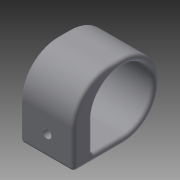
# Autodesk Inventor part: LoopD
Saved by Autodesk Inventor 2014 (Build 180170000, 170)
## iProperties
Created: 2014-06-16
Part Number: LoopD
Material: Generisch
Document SubType Name: Modeling
Designer: g.schardt
Density: 1 g/cm^3
Appearance: Vorgabe
Author: g.schardt
Autodesk Inventor part; units mm, degrees
ref_plane "YZ Plane" through (0, 0, 0) normal (1, 0, 0) x (0, 1, 0)
ref_plane "XZ Plane" through (0, 0, 0) normal (0, 1, 0) x (-1, 0, 0)
ref_plane "XY Plane" through (0, 0, 0) normal (0, 0, 1) x (1, 0, 0)
sketch "Skizze1" plane through (0, 0, 0) normal (1, 0, 0) x (0, 1, 0)
  line L0 (-21, -18) -> (21, -18)
  line L1 (21, -18) -> (21, 18)
  line L2 (21, 18) -> (-21, 18)
  line L3 (-21, 18) -> (-21, -18)
  line L4 (-21, -18) -> (21, 18) construction
  line L5 (21, -18) -> (-21, 18) construction
  point P0 (0, 0)
  dimension "d0" = 42
  dimension "d1" = 36
  constraints: 12 end point, 2 midpoint, 2 parallel, 1 horizontal, 1 perpendicular
  measures "d0" distance of L2.end L1.end
  measures "d1" distance of L1.end L0.end
extrude "Extrusion1" add sketch "Skizze1" along normal blind 26
sketch "Skizze2" plane through (26, 0, 0) normal (1, 0, 0) x (0, 0, -1)
  line L0 (18, 21) -> (-18, 21) projected
  line L1 (-18, 21) -> (-18, -21) projected
  line L2 (-15, 18) -> (15, 18)
  line L3 (15, 18) -> (15, -12)
  line L4 (15, -12) -> (-15, -12)
  line L5 (-15, -12) -> (-15, 18)
  point P0 (0, 0)
  dimension "d4" = 30
  dimension "d5" = 30
  dimension "d6" = 3
  dimension "d7" = 3
  constraints: 8 end point, 2 parallel, 1 horizontal, 1 perpendicular
  measures "d4" distance of L2.start L2.end
  measures "d5" distance between parallel lines of L4 L2
  measures "d6" distance between parallel lines of L0 L2
  measures "d7" distance between parallel lines of L1 L5
extrude "Extrusion2" cut sketch "Skizze2" against normal through all
fillet "Rundung1" radius 15 1 edges at (13, 18, -15)
fillet "Rundung2" radius 15 1 edges at (13, 18, 15)
fillet "Rundung3" radius 18 2 edges at (13, 21, 18) (13, 21, -18)
ref_plane "Arbeitsebene1" through (0, -18, -18) normal (0, -1, 0) x (1, 0, 0)
ref_plane "Arbeitsebene2" through (0, -14.8, -18) normal (0, -1, 0) x (1, 0, 0)
sketch "Skizze3" plane through (0, -21, -18) normal (0, -1, 0) x (1, 0, 0)
  line L0 (0, 36) -> (0, 0) projected
  line L1 (0, 0) -> (26, 0) projected
  line L2 (3, 0) -> (23, 0)
  line L3 (23, 0) -> (23, 17)
  line L4 (23, 17) -> (3, 17)
  line L5 (3, 17) -> (3, 0)
  point P0 (0, 18)
  dimension "d15" = 20
  dimension "d16" = 17
  dimension "d17" = 3
  constraints: 8 end point, 2 parallel, 1 horizontal, 1 perpendicular, 1 point on line
  measures "d15" distance of L4.end L3.end
  measures "d16" distance of L3.end L2.end
  measures "d17" distance between parallel lines of L0 L5
extrude "Extrusion3" cut sketch "Skizze3" against normal up to surface (3.2 mm away) from surface at -3
fillet "Rundung4" radius 9 2 edges at (3, -16.4, -1) (23, -16.4, -1)
sketch "Skizze4" plane through (26, -12, 15) normal (0, 1, 0) x (1, 0, 0)
  line L0 (0, 30) -> (0, 0) projected
  line L1 (-26, -3) -> (0, -3) projected
  line L2 (-3, 33) -> (-23, 33) projected
  point P0 (-26, 15)
  point P1 (-13, 23)
  dimension "d29" = 13
  dimension "d31" = 10
  measures "d29" distance from line of L0 point (-13, 23)
  measures "d31" distance from line of L2 point (-13, 23)
hole "Bohrung1" at (13, -12, -8) direction (0, -1, 0) diameter 4.2 end through all countersink diameter 7.5 countersink angle 90
fillet "Rundung10" radius 15 1 edges at (13, -12, 15)
fillet "Rundung11" radius 18 1 edges at (13, -21, 18)
fillet "Rundung12" radius 1.5 29 edges at (26, -8.9999, -18) (26, 0, 18) (26, -15.7279, 12.7279) (26, -21, -9) (26, 15.728, 12.728) (26, 21, 0) (26, 15.728, -12.728) (26, -12, -7.5) (26, -4.5, -15) (26, 3, 15) (26, -7.6066, 10.6066) (26, 13.6066, 10.6066) (26, 18, 0.0001) (26, 13.6066, -10.6066) (0, -21, -9) (0, 0, 18) (0, 15.728, 12.728) (0, 21, 0) (0, 15.728, -12.728) (0, -8.9999, -18) (0, -15.7279, 12.7279) (0, -4.5, -15) (0, -12, -7.5) (0, 3, 15) (0, -7.6066, 10.6066) (0, 13.6066, 10.6066) (0, 18, 0.0001) (0, 13.6066, -10.6066) (13, -12, -15)
fillet "Rundung13" radius 1.5 3 edges at (25.5607, -20.5607, -17.5607) (0.4393, -20.5607, -17.5607) (13, -21, -18)
chamfer "Fase1" distance 0.5 angle 45 4 edges at (13, -14.8, -18) (23, -16.4, -18) (13, -18, -18) (3, -16.4, -18)
